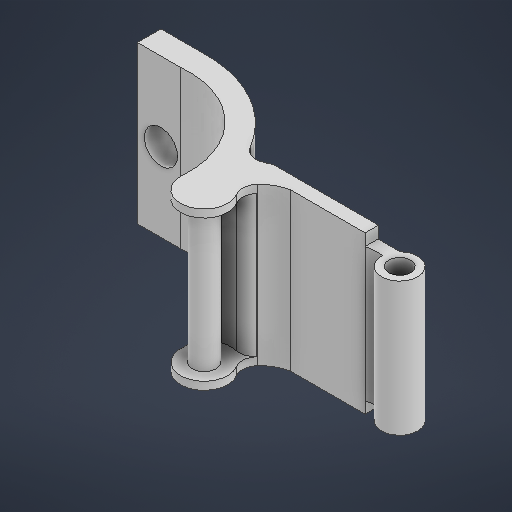
# Autodesk Inventor part: arm_1
Saved by Autodesk Inventor 2027 (Build 310192060, 192F)
## iProperties
Created: 2026-05-15
Part Number: arm_1
Material: Ogólny
Document SubType Name: Modeling
Designer: User
Density: 1 g/cm^3
Appearance: Domyślna
Mass: 0.967424 g
Surface Area: 12.9312 cm^2
Volume: 0.967424 cm^3
Author: User
Autodesk Inventor part; units mm, degrees
ref_plane "YZ Plane" through (0, 0, 0) normal (1, 0, 0) x (0, 1, 0)
ref_plane "XZ Plane" through (0, 0, 0) normal (0, 1, 0) x (-1, 0, 0)
ref_plane "XY Plane" through (0, 0, 0) normal (0, 0, 1) x (1, 0, 0)
sketch "Szkic1" plane through (0, 0, 0) normal (0, 1, 0) x (-1, 0, 0)
  circle A0 centre (0, 0) radius 2.3
  circle A1 centre (0, 0) radius 1.4
  arc A2 (1.4, 0) -> (4.4, 0) centre (2.9, 6.8374) ccw
  line L0 (0, -1.4) -> (4.4, -1.4)
  line L1 (4.4, 0) -> (4.4, -1.4)
  point P0 (1.8248, -1.4)
  point P1 (2.2959, -0.1365)
  dimension "d0" = 4.6
  dimension "d1" = 2.8
  dimension "d2" = 3
  dimension "d3" = 7
  constraints: 4 end point, 4 point on circle, 3 centre point, 2 coincident, 1 horizontal, 1 vertical
  measures "d0" diameter of A0
  measures "d1" diameter of A1
  measures "d2" distance of A1.start L1.start
  measures "d3" radius of A2
extrude "Wyciągnięcie proste1" add sketch "Szkic1" along normal blind 17 contours A0 A2 A1 L0 | L0 A1 A2 A0 | A0 A2 L1 L0
ref_plane "Płaszczyzna konstrukcyjna1" through (0, 8.5, 0) normal (0, 1, 0) x (1, 0, 0)
sketch "Szkic2" plane through (0, 8.5, 0) normal (0, 1, 0) x (1, 0, 0)
  arc A0 (-2.2959, 0.1365) -> (-4.4, 0) centre (-2.9, -6.8374) ccw projected
  line L0 (-4.4, 0) -> (-19.4, 0)
  line L1 (-19.4, 0) -> (-19.4, 1.7)
  line L2 (-19.4, 1.7) -> (-4.4, 1.7)
  line L3 (-4.4, 1.7) -> (-4.4, 0)
  line L4 (-19.4, 0) -> (-19.4, -4) construction
  line L5 (-19.4, -4) -> (-19.4, -5.5) construction
  circle A1 centre (-19.4, -5.5) radius 1.5
  circle A2 centre (-19.4, -5.5) radius 3
  arc A3 (-11.9, 0) -> (-17.6064, -3.0952) centre (-12.9148, -4.9368) ccw
  line L6 (-19.4, -2.5) -> (-19.4, 1.7)
  line L7 (-19.4, -5.5) -> (-34.4, -5.5) construction
  line L8 (-34.4, -5.5) -> (-34.4, 6.5) construction
  line L9 (-34.4, 6.5) -> (-39.4, 6.5)
  line L10 (-39.4, 6.5) -> (-39.4, 9.5)
  line L11 (-39.4, 9.5) -> (-34.4, 9.5)
  line L12 (-34.4, 9.5) -> (-34.4, 6.5)
  arc A4 (-19.4, -2.5) -> (-34.4, 9.5) centre (-34.0976, -5.497) ccw
  arc A5 (-22.4, -5.5) -> (-34.4, 6.5) centre (-33.3497, -4.4497) ccw
  circle A6 centre (-19.4, -5.5) radius 2.2
  point P0 (0, 0)
  point P1 (-19.4, 0)
  point P2 (-13.9296, 0)
  point P3 (-22.3662, -5.0508)
  dimension "d14" = 15
  dimension "d16" = 1.7
  dimension "d28" = 4
  dimension "d29" = 1.5
  dimension "d30" = 6
  dimension "d31" = 15
  dimension "d32" = 12
  dimension "d33" = 5
  dimension "d34" = 3
  dimension "d35" = 15
  dimension "d36" = 11
  dimension "d38" = 4.4
  constraints: 26 end point, 9 point on circle, 5 centre point, 4 parallel, 3 coincident, 3 horizontal, 3 perpendicular, 2 vertical, 1 collinear, 1 midpoint, 1 point on line, 1 vertical alignment, 2 other
  measures "d14" distance of L1.end L2.end
  measures "d16" distance of L0.end L1.end
  measures "d28" distance of L0.end L4.end
  measures "d29" distance of L4.end L5.end
  measures "d30" diameter of A2
  measures "d31" distance of L7.start L7.end
  measures "d32" distance of L7.end L8.end
  measures "d33" distance of L10.end L11.end
  measures "d34" distance of L9.end L10.end
  measures "d35" radius of A4
  measures "d36" radius of A5
  measures "d38" diameter of A6
extrude "Wyciągnięcie proste2" add sketch "Szkic2" along normal mid plane 20 contours L0 A3 L1 L2 L3 | L0 A3 | A3 A2 L6 L0 | A2 A5 | A2 A5 L12 A4 | A5 A2 | L12 L9 L10 L11 | A1 | A6
offset faces "Rozmiar1" outward 0.25 faces at (-2.6832, 5.6667, -1.4)
fillet "Zaokrąglenie1" radius 2 2 edges at (-19.4, 8.5, 2.5) (-19.4, 8.5, -1.7)
fillet "Zaokrąglenie2" radius 2 1 edges at (-17.6064, 8.5, 3.0952)
ref_plane "Płaszczyzna konstrukcyjna2" through (0, 13.5, 0) normal (0, 1, 0) x (1, 0, 0)
sketch "Szkic3" plane through (0, 13.5, 0) normal (0, 1, 0) x (1, 0, 0)
  arc A0 (-22.3662, -5.0508) -> (-16.8477, -3.9233) centre (-19.4, -5.5) ccw projected
  circle A1 centre (-19.4, -5.5) radius 1.5
  circle A2 centre (-19.4, -5.5) radius 3.3976
  point P0 (0, 0)
  point P1 (-22.4, -5.5)
  dimension "d41" = 3
  constraints: 2 centre point, 2 coincident
  measures "d41" diameter of A1
extrude "Wyciągnięcie proste3" cut sketch "Szkic3" along normal blind 4 and the other way blind 14
fillet "Zaokrąglenie3" radius 2 3 edges at (-17.1443, 15.5, 2.9592) (-17.1443, 6.5, 2.9592) (-22.3665, 8.5, 3.8435)
sketch "Szkic4" plane through (-34.4, 18.5, -9.5) normal (0, 0, -1) x (-1, 0, 0)
  line L0 (5, -20) -> (5, 0) projected
  line L1 (0, -20) -> (5, -20) projected
  line L2 (5, 0) -> (0, 0)
  line L3 (0, 0) -> (0, -20)
  line L4 (0, -20) -> (5, -20)
  line L5 (5, -20) -> (5, 0)
  line L6 (5, 0) -> (0, 0)
  line L7 (0, 0) -> (0, -10)
  line L8 (0, -10) -> (5, -10)
  line L9 (5, -10) -> (5, 0)
  line L10 (5, -10) -> (0, -10)
  line L11 (0, -10) -> (0, -20)
  line L12 (0, -20) -> (5, -20)
  line L13 (5, -20) -> (5, -10)
  circle A0 centre (2.5, -10) radius 2.125
  point P0 (-34.4, -18.5)
  dimension "d45" = 4.25
  dimension "d49" = 2.5
  dimension "d50" = 10
  constraints: 24 end point, 6 parallel, 3 horizontal, 3 perpendicular, 1 centre point, 1 midpoint
  measures "d45" diameter of A0
  measures "d49" distance from line of L3 A0.centre
  measures "d50" distance from line of L2 A0.centre
extrude "Wyciągnięcie proste4" cut sketch "Szkic4" against normal blind 8 contours A0 L8 | L8 A0
move faces "Przesuń1" translate (-0.5, 0, 0) faces at (-39.4, 11.8333, -7.5)
equation "\"d17\" = Height"
equation "\"Height\" = 20"
equation "\"d4\" = 6"
equation "\"d8\" = 1"
equation "\"d9\" = 1"
equation "\"d10\" = 150deg"
equation "\"d11\" = 1"
equation "\"d15\" = 2.02977"
equation "\"d21\" = 0"
equation "\"d23\" = 3"
equation "\"d25\" = 0"
equation "\"d27\" = 2"
equation "\"Joint_shaft\" = 18"
equation "\"Joint_diam\" = 3"
equation "\"d12\" = Joint_diam"
equation "\"d24\" = Joint_shaft"
